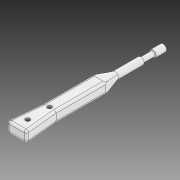
# Autodesk Inventor part: 6103_Bulb Arm_Microcentrifuge-tube
Saved by Autodesk Inventor 2021 (Build 250183000, 183)
## iProperties
Created: 2019-10-22
Part Number: 6103_Bulb Arm_Microcentrifuge-tube
Material: ABS Plastic
Document SubType Name: Modeling
Designer: RFLab
Density: 1.06 g/cm^3
Appearance: Smooth - White
Author: RFLab
Autodesk Inventor part; units mm, degrees
ref_plane "YZ Plane" through (0, 0, 0) normal (1, 0, 0) x (0, 1, 0)
ref_plane "XZ Plane" through (0, 0, 0) normal (0, 1, 0) x (-1, 0, 0)
ref_plane "XY Plane" through (0, 0, 0) normal (0, 0, 1) x (1, 0, 0)
sketch "Sketch8" plane through (0, 0, 0) normal (0, 0, 1) x (1, 0, 0)
  line L0 (-5.9, -5) -> (5.9, -5)
  line L1 (5.9, -5) -> (5.9, 5)
  line L2 (5.9, 5) -> (-5.9, 5)
  line L3 (-5.9, 5) -> (-5.9, -5)
  line L4 (-5.9, -5) -> (5.9, 5) construction
  line L5 (5.9, -5) -> (-5.9, 5) construction
  point P0 (0, 0)
  dimension "d41" = 11.8
  dimension "d42" = 10
  constraints: 12 end point, 2 midpoint, 2 parallel, 1 horizontal, 1 perpendicular
  measures "d41" distance of L2.end L1.end
  measures "d42" distance of L1.end L0.end
extrude "Extrusion8" add sketch "Sketch8" along normal blind 75
sketch "Sketch9" plane through (0, 0, 0) normal (0, 0, -1) x (-1, 0, 0)
  line L0 (5.9, 5) -> (5.9, -5) projected
  circle A0 centre (0, 0) radius 3
  point P0 (0, 0)
  point P1 (5.9, 0)
  dimension "d45" = 6
  constraints: 1 centre point, 1 horizontal alignment, 1 midpoint
  measures "d45" diameter of A0
extrude "Extrusion9" add sketch "Sketch9" along normal blind 59
sketch "Sketch10" plane through (0, 0, 0) normal (0, 0, -1) x (-1, 0, 0)
  line L0 (5.9, -5) -> (-5.9, -5) projected
  line L1 (5.9, 5) -> (5.9, -5) projected
  line L2 (-5.9, 5) -> (5.9, 5) projected
  line L3 (-5.9, -5) -> (-5.9, 5) projected
ref_plane "Work Plane2" through (0, 0, -15) normal (0, 0, -1) x (-1, 0, 0)
sketch "Sketch11" plane through (0, 0, -15) normal (0, 0, -1) x (-1, 0, 0)
  circle A0 centre (0, 0) radius 3 projected
  point P0 (0, 0)
loft "Loft3" add profiles "Sketch10", "Sketch11"
sketch "Sketch14" plane through (-5.9, 5, 75) normal (0, 1, 0) x (1, 0, 0)
  line L0 (11.8, 0) -> (0, 0) projected
  line L1 (0, 0) -> (11.8, 0) projected
  line L2 (5.9, 0) -> (5.9, 75)
  point P0 (5.9, 10)
  point P1 (5.9, 30)
  dimension "d64" = 10
  dimension "d65" = 30
  constraints: 2 end point, 2 point on line, 1 midpoint, 1 perpendicular
  measures "d64" distance from line of L0 point (5.9, 10)
  measures "d65" distance from line of L0 point (5.9, 30)
hole "Hole1" at (0, 5, 65) at (0, 5, 45) direction (0, -1, 0) diameter 4 end through all
sketch "Sketch15" plane through (-5.9, -5, 75) normal (0, -1, 0) x (1, 0, 0)
  circle A0 centre (5.9, -10) radius 2 projected
  circle A1 centre (5.9, -30) radius 2 projected
  line L0 (0, -75) -> (11.8, -75) projected
  line L1 (11.8, -75) -> (11.8, 0) projected
  line L2 (0, 0) -> (11.8, 0) projected
  line L3 (0, -75) -> (0, 0) projected
  line L4 (11.8, 0) -> (14.7, 0)
  line L5 (14.7, 0) -> (11.8, -30)
  line L6 (11.8, -75) -> (11.8, 0) projected
  line L7 (0, -75) -> (0, 0) projected
  line L8 (0, 0) -> (-2.9, 0)
  line L9 (-2.9, 0) -> (0, -30)
  point P0 (5.9, -75)
  dimension "d73" = 2.9
  dimension "d74" = 2.9
  constraints: 8 end point, 3 point on line, 2 horizontal alignment, 1 horizontal
  measures "d73" distance of L2.start L8.end
  measures "d74" distance of L1.end L4.end
extrude "Extrusion12" add sketch "Sketch15" against normal up to surface (10 mm away) contours L9 L8 L3 | L1 L4 L5
fillet "Fillet4" radius 2 12 edges at (-8.8, 0, 75) (8.8, 0, 75) (-7.35, 5, 60) (0, 5, 75) (7.35, 5, 60) (-5.9, 5, 22.5) (-5.9, -5, 22.5) (5.9, -5, 22.5) (7.35, -5, 60) (0, -5, 75) (5.9, 5, 22.5) (-7.35, -5, 60)
sketch "Sketch16" plane through (0, 0, 0) normal (1, 0, 0) x (0, 1, 0)
  line L0 (-3, -59) -> (3, -59) projected
  line L1 (-1.9396, -15) -> (-1.9396, -15) projected
  line L2 (-1.9396, -15) -> (1.9396, -15) projected
  line L3 (1.9396, -15) -> (1.9396, -15) projected
  line L4 (1.9396, -15) -> (-1.9396, -15) projected
  line L5 (-3, -59) -> (3, -59) projected
  line L6 (3, -15) -> (3, -59) projected
  line L7 (-3, -59) -> (3, -59)
  line L8 (3, -59) -> (3, -38.8034)
  line L9 (3, -38.8034) -> (-3, -38.8034)
  line L10 (-3, -38.8034) -> (-3, -59)
  line L11 (3, -38.5075) -> (2, -38.5075)
  line L12 (2, -38.5075) -> (2, -49.5075)
  line L13 (2, -49.5075) -> (3, -49.5075)
  line L14 (3, -49.5075) -> (3, -38.5075)
  line L15 (0, -70.8) -> (0, 11.8) projected
  point P0 (0, 0)
  dimension "d78" = 1
  dimension "d79" = 11
  constraints: 16 end point, 4 parallel, 2 horizontal, 2 perpendicular, 2 point on line
  measures "d78" distance of L13.end L12.end
  measures "d79" distance of L12.end L11.end
revolve "Revolution1" cut sketch "Sketch16" angle 360 about axis through (0, 0, -10) along (0, 0, 1) contours L13 L12 L9 L6 | L12 L11 L6 L9
sketch "Sketch17" plane through (0, 0, 0) normal (0, 1, 0) x (-1, 0, 0)
  line L0 (-2.2887, -15) -> (2.2887, -15) projected
  line L1 (2.2887, -15) -> (2.2887, -15) projected
  line L2 (2.2887, -15) -> (-2.2887, -15) projected
  line L3 (-2.2887, -15) -> (-2.2887, -15) projected
  line L4 (3, -38.5075) -> (-3, -38.5075) projected
  line L5 (-3, -59) -> (3, -59) projected
  line L6 (3, -34) -> (-3, -34)
  line L7 (-3, -34) -> (-3, -59)
  line L8 (-3, -59) -> (3, -59)
  line L9 (3, -59) -> (3, -34)
  point P0 (0, 0)
  dimension "d81" = 25
  constraints: 8 end point, 2 parallel, 1 horizontal, 1 perpendicular, 1 point on line
  measures "d81" distance of L8.end L6.start
sketch "Sketch18" plane through (0, 0, 0) normal (0, 1, 0) x (1, 0, 0)
  circle A0 centre (0, 55) radius 1.75
  line L0 (-3, 59) -> (3, 59) projected
  point P0 (0, 0)
  dimension "d84" = 3.5
  dimension "d85" = 4
  constraints: 1 centre point
  measures "d84" diameter of A0
  measures "d85" distance from line of L0 A0.centre
sketch "Sketch19" plane through (3, 0, -34) normal (0, 0, -1) x (-1, 0, 0)
  circle A0 centre (3, 0) radius 0.9
  dimension "d88" = 1.8
  constraints: 1 centre point, 1 coincident
  measures "d88" diameter of A0
sketch "Sketch20" plane through (0, 0, -34) normal (0, 0, -1) x (-1, 0, 0)
  circle A0 centre (0, 0) radius 1.5
  dimension "d91" = 3
  constraints: 1 centre point, 1 coincident, 1 horizontal alignment
  measures "d91" diameter of A0
sketch "Sketch21" plane through (0, 0, 0) normal (0, 1, 0) x (1, 0, 0)
  arc A0 (0.9, 39.0193) -> (1.2, 38.3052) centre (1.9, 39.0193) ccw projected
  arc A1 (1.5, 37.591) -> (1.2, 38.3052) centre (0.5, 37.591) ccw projected
  line L0 (1.5, 37.591) -> (1.5, 35) projected
  line L1 (3, 35) -> (1.5, 35) projected
  line L2 (3, 35) -> (3, 37.7755) projected
  arc A2 (3, 37.7755) -> (2.5, 38.6415) centre (2, 37.7755) ccw projected
  arc A3 (2, 39.5075) -> (2.5, 38.6415) centre (3, 39.5075) ccw projected
  line L3 (2, 48.5075) -> (2, 39.5075) projected
  arc A4 (3, 49.5075) -> (2, 48.5075) centre (3, 48.5075) ccw projected
  line L4 (3, 49.5075) -> (3, 59) projected
  line L5 (-3, 59) -> (3, 59) projected
  line L6 (-3, 49.5075) -> (-3, 59) projected
  arc A5 (-2, 48.5075) -> (-3, 49.5075) centre (-3, 48.5075) ccw projected
  line L7 (-2, 39.5075) -> (-2, 48.5075) projected
  arc A6 (-2.5, 38.6415) -> (-2, 39.5075) centre (-3, 39.5075) ccw projected
  arc A7 (-2.5, 38.6415) -> (-3, 37.7755) centre (-2, 37.7755) ccw projected
  line L8 (-3, 35) -> (-3, 37.7755) projected
  line L9 (-1.5, 35) -> (-3, 35) projected
  line L10 (-1.5, 35) -> (-1.5, 37.591) projected
  arc A8 (-1.2, 38.3052) -> (-1.5, 37.591) centre (-0.5, 37.591) ccw projected
  arc A9 (-1.2, 38.3052) -> (-0.9, 39.0193) centre (-1.9, 39.0193) ccw projected
  line L11 (-0.9, 39.0193) -> (-0.9, 53.0119) projected
  arc A10 (1.2091, 53.7349) -> (-1.2091, 53.7349) centre (0, 55) ccw projected
  line L12 (0.9, 53.0119) -> (0.9, 39.0193) projected
  arc A11 (1.2091, 53.7349) -> (-1.2091, 53.7349) centre (0, 55) ccw projected
  line L13 (-1.75, 55) -> (-3, 55)
  line L14 (1.75, 55) -> (3.2552, 55)
  point P0 (0, 0)
  point P1 (3, 55)
  constraints: 4 end point, 3 point on line, 2 point on circle, 1 horizontal, 1 line through centre, 2 other
sketch "Sketch22" plane through (0, 0, -59) normal (0, 0, -1) x (-1, 0, 0)
  arc A0 (-3, 0) -> (3, 0) centre (0, 0) ccw projected
  circle A1 centre (0, 0) radius 0.5 projected
  circle A2 centre (0, 0) radius 3
  arc A3 (-3, 0) -> (3, 0) centre (0, 0) ccw projected
  line L0 (3, 0) -> (3, 1.5) projected
  line L1 (-3, 1.5) -> (3, 1.5) projected
  line L2 (-3, 0) -> (-3, 1.5) projected
  point P0 (-2.5981, 1.5)
  point P1 (3, 0)
  point P2 (2.5981, 1.5)
  constraints: 1 centre point, 1 coincident, 1 concentric
equation "\"d74\" = d73"
body "Solid2"
